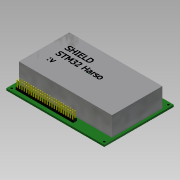
# Autodesk Inventor part: shieldstm
Saved by Autodesk Inventor 2015 SP1 (Build 190203100, 203)
## iProperties
Created: 2015-02-03
Part Number: shieldstm
Material: Generic
Document SubType Name: Modeling
Designer: Rafi Kurnia Putra
Density: 1 g/cm^3
Appearance: Smooth - Yellow
Mass: 140.996 g
Surface Area: 307.054 cm^2
Volume: 140.996 cm^3
Author: Rafi Kurnia Putra
Autodesk Inventor part; units mm, degrees
ref_plane "YZ Plane" through (0, 0, 0) normal (1, 0, 0) x (0, 1, 0)
ref_plane "XZ Plane" through (0, 0, 0) normal (0, 1, 0) x (-1, 0, 0)
ref_plane "XY Plane" through (0, 0, 0) normal (0, 0, 1) x (1, 0, 0)
sketch "Sketch1" plane through (0, 0, 0) normal (0, 1, 0) x (-1, 0, 0)
  line L0 (53.5965, 37.9955) -> (-53.5965, 37.9955)
  line L1 (-53.5965, 37.9955) -> (-53.5965, -37.9955)
  line L2 (-53.5965, -37.9955) -> (53.5965, -37.9955)
  line L3 (53.5965, -37.9955) -> (53.5965, 37.9955)
  line L4 (53.5965, 37.9955) -> (-53.5965, -37.9955) construction
  line L5 (-53.5965, 37.9955) -> (53.5965, -37.9955) construction
  circle A0 centre (50.5965, 34.9955) radius 1
  circle A1 centre (50.5965, -34.9955) radius 1
  circle A2 centre (-50.5965, 34.9955) radius 1
  circle A3 centre (-50.5965, -34.9955) radius 1
  line L6 (46.185, 33.9325) -> (45.392, 33.9325)
  line L7 (45.392, 33.9325) -> (45.392, 33.1485)
  line L8 (45.392, 33.1485) -> (46.185, 33.1485)
  line L9 (46.185, 33.1485) -> (46.185, 33.9325)
  line L10 (46.185, 33.9325) -> (45.392, 33.1485) construction
  line L11 (45.392, 33.9325) -> (46.185, 33.1485) construction
  line L12 (43.665, 33.9325) -> (42.872, 33.9325)
  line L13 (42.872, 33.9325) -> (42.872, 33.1485)
  line L14 (42.872, 33.1485) -> (43.665, 33.1485)
  line L15 (43.665, 33.1485) -> (43.665, 33.9325)
  line L16 (41.145, 33.9325) -> (40.352, 33.9325)
  line L17 (40.352, 33.9325) -> (40.352, 33.1485)
  line L18 (40.352, 33.1485) -> (41.145, 33.1485)
  line L19 (41.145, 33.1485) -> (41.145, 33.9325)
  line L20 (38.625, 33.9325) -> (37.832, 33.9325)
  line L21 (37.832, 33.9325) -> (37.832, 33.1485)
  line L22 (37.832, 33.1485) -> (38.625, 33.1485)
  line L23 (38.625, 33.1485) -> (38.625, 33.9325)
  line L24 (36.105, 33.9325) -> (35.312, 33.9325)
  line L25 (35.312, 33.9325) -> (35.312, 33.1485)
  line L26 (35.312, 33.1485) -> (36.105, 33.1485)
  line L27 (36.105, 33.1485) -> (36.105, 33.9325)
  line L28 (33.585, 33.9325) -> (32.792, 33.9325)
  line L29 (32.792, 33.9325) -> (32.792, 33.1485)
  line L30 (32.792, 33.1485) -> (33.585, 33.1485)
  line L31 (33.585, 33.1485) -> (33.585, 33.9325)
  line L32 (31.065, 33.9325) -> (30.272, 33.9325)
  line L33 (30.272, 33.9325) -> (30.272, 33.1485)
  line L34 (30.272, 33.1485) -> (31.065, 33.1485)
  line L35 (31.065, 33.1485) -> (31.065, 33.9325)
  line L36 (28.545, 33.9325) -> (27.752, 33.9325)
  line L37 (27.752, 33.9325) -> (27.752, 33.1485)
  line L38 (27.752, 33.1485) -> (28.545, 33.1485)
  line L39 (28.545, 33.1485) -> (28.545, 33.9325)
  line L40 (26.025, 33.9325) -> (25.232, 33.9325)
  line L41 (25.232, 33.9325) -> (25.232, 33.1485)
  line L42 (25.232, 33.1485) -> (26.025, 33.1485)
  line L43 (26.025, 33.1485) -> (26.025, 33.9325)
  line L44 (23.505, 33.9325) -> (22.712, 33.9325)
  line L45 (22.712, 33.9325) -> (22.712, 33.1485)
  line L46 (22.712, 33.1485) -> (23.505, 33.1485)
  line L47 (23.505, 33.1485) -> (23.505, 33.9325)
  line L48 (20.985, 33.9325) -> (20.192, 33.9325)
  line L49 (20.192, 33.9325) -> (20.192, 33.1485)
  line L50 (20.192, 33.1485) -> (20.985, 33.1485)
  line L51 (20.985, 33.1485) -> (20.985, 33.9325)
  line L52 (18.465, 33.9325) -> (17.672, 33.9325)
  line L53 (17.672, 33.9325) -> (17.672, 33.1485)
  line L54 (17.672, 33.1485) -> (18.465, 33.1485)
  line L55 (18.465, 33.1485) -> (18.465, 33.9325)
  line L56 (15.945, 33.9325) -> (15.152, 33.9325)
  line L57 (15.152, 33.9325) -> (15.152, 33.1485)
  line L58 (15.152, 33.1485) -> (15.945, 33.1485)
  line L59 (15.945, 33.1485) -> (15.945, 33.9325)
  line L60 (13.425, 33.9325) -> (12.632, 33.9325)
  line L61 (12.632, 33.9325) -> (12.632, 33.1485)
  line L62 (12.632, 33.1485) -> (13.425, 33.1485)
  line L63 (13.425, 33.1485) -> (13.425, 33.9325)
  line L64 (10.905, 33.9325) -> (10.112, 33.9325)
  line L65 (10.112, 33.9325) -> (10.112, 33.1485)
  line L66 (10.112, 33.1485) -> (10.905, 33.1485)
  line L67 (10.905, 33.1485) -> (10.905, 33.9325)
  line L68 (8.385, 33.9325) -> (7.592, 33.9325)
  line L69 (7.592, 33.9325) -> (7.592, 33.1485)
  line L70 (7.592, 33.1485) -> (8.385, 33.1485)
  line L71 (8.385, 33.1485) -> (8.385, 33.9325)
  line L72 (5.865, 33.9325) -> (5.072, 33.9325)
  line L73 (5.072, 33.9325) -> (5.072, 33.1485)
  line L74 (5.072, 33.1485) -> (5.865, 33.1485)
  line L75 (5.865, 33.1485) -> (5.865, 33.9325)
  line L76 (3.345, 33.9325) -> (2.552, 33.9325)
  line L77 (2.552, 33.9325) -> (2.552, 33.1485)
  line L78 (2.552, 33.1485) -> (3.345, 33.1485)
  line L79 (3.345, 33.1485) -> (3.345, 33.9325)
  line L80 (0.825, 33.9325) -> (0.032, 33.9325)
  line L81 (0.032, 33.9325) -> (0.032, 33.1485)
  line L82 (0.032, 33.1485) -> (0.825, 33.1485)
  line L83 (0.825, 33.1485) -> (0.825, 33.9325)
  line L84 (-1.695, 33.9325) -> (-2.488, 33.9325)
  line L85 (-2.488, 33.9325) -> (-2.488, 33.1485)
  line L86 (-2.488, 33.1485) -> (-1.695, 33.1485)
  line L87 (-1.695, 33.1485) -> (-1.695, 33.9325)
  line L88 (-4.215, 33.9325) -> (-5.008, 33.9325)
  line L89 (-5.008, 33.9325) -> (-5.008, 33.1485)
  line L90 (-5.008, 33.1485) -> (-4.215, 33.1485)
  line L91 (-4.215, 33.1485) -> (-4.215, 33.9325)
  line L92 (-6.735, 33.9325) -> (-7.528, 33.9325)
  line L93 (-7.528, 33.9325) -> (-7.528, 33.1485)
  line L94 (-7.528, 33.1485) -> (-6.735, 33.1485)
  line L95 (-6.735, 33.1485) -> (-6.735, 33.9325)
  line L96 (-9.255, 33.9325) -> (-10.048, 33.9325)
  line L97 (-10.048, 33.9325) -> (-10.048, 33.1485)
  line L98 (-10.048, 33.1485) -> (-9.255, 33.1485)
  line L99 (-9.255, 33.1485) -> (-9.255, 33.9325)
  line L100 (-11.775, 33.9325) -> (-12.568, 33.9325)
  line L101 (-12.568, 33.9325) -> (-12.568, 33.1485)
  line L102 (-12.568, 33.1485) -> (-11.775, 33.1485)
  line L103 (-11.775, 33.1485) -> (-11.775, 33.9325)
  line L104 (-14.295, 33.9325) -> (-15.088, 33.9325)
  line L105 (-15.088, 33.9325) -> (-15.088, 33.1485)
  line L106 (-15.088, 33.1485) -> (-14.295, 33.1485)
  line L107 (-14.295, 33.1485) -> (-14.295, 33.9325)
  line L108 (46.185, 31.4325) -> (45.392, 31.4325)
  line L109 (45.392, 31.4325) -> (45.392, 30.6485)
  line L110 (45.392, 30.6485) -> (46.185, 30.6485)
  line L111 (46.185, 30.6485) -> (46.185, 31.4325)
  line L112 (43.665, 31.4325) -> (42.872, 31.4325)
  line L113 (42.872, 31.4325) -> (42.872, 30.6485)
  line L114 (42.872, 30.6485) -> (43.665, 30.6485)
  line L115 (43.665, 30.6485) -> (43.665, 31.4325)
  line L116 (41.145, 31.4325) -> (40.352, 31.4325)
  line L117 (40.352, 31.4325) -> (40.352, 30.6485)
  line L118 (40.352, 30.6485) -> (41.145, 30.6485)
  line L119 (41.145, 30.6485) -> (41.145, 31.4325)
  line L120 (38.625, 31.4325) -> (37.832, 31.4325)
  line L121 (37.832, 31.4325) -> (37.832, 30.6485)
  line L122 (37.832, 30.6485) -> (38.625, 30.6485)
  line L123 (38.625, 30.6485) -> (38.625, 31.4325)
  line L124 (36.105, 31.4325) -> (35.312, 31.4325)
  line L125 (35.312, 31.4325) -> (35.312, 30.6485)
  line L126 (35.312, 30.6485) -> (36.105, 30.6485)
  line L127 (36.105, 30.6485) -> (36.105, 31.4325)
  line L128 (33.585, 31.4325) -> (32.792, 31.4325)
  line L129 (32.792, 31.4325) -> (32.792, 30.6485)
  line L130 (32.792, 30.6485) -> (33.585, 30.6485)
  line L131 (33.585, 30.6485) -> (33.585, 31.4325)
  line L132 (31.065, 31.4325) -> (30.272, 31.4325)
  line L133 (30.272, 31.4325) -> (30.272, 30.6485)
  line L134 (30.272, 30.6485) -> (31.065, 30.6485)
  line L135 (31.065, 30.6485) -> (31.065, 31.4325)
  line L136 (28.545, 31.4325) -> (27.752, 31.4325)
  line L137 (27.752, 31.4325) -> (27.752, 30.6485)
  line L138 (27.752, 30.6485) -> (28.545, 30.6485)
  line L139 (28.545, 30.6485) -> (28.545, 31.4325)
  line L140 (26.025, 31.4325) -> (25.232, 31.4325)
  line L141 (25.232, 31.4325) -> (25.232, 30.6485)
  line L142 (25.232, 30.6485) -> (26.025, 30.6485)
  line L143 (26.025, 30.6485) -> (26.025, 31.4325)
  line L144 (23.505, 31.4325) -> (22.712, 31.4325)
  line L145 (22.712, 31.4325) -> (22.712, 30.6485)
  line L146 (22.712, 30.6485) -> (23.505, 30.6485)
  line L147 (23.505, 30.6485) -> (23.505, 31.4325)
  line L148 (20.985, 31.4325) -> (20.192, 31.4325)
  line L149 (20.192, 31.4325) -> (20.192, 30.6485)
  line L150 (20.192, 30.6485) -> (20.985, 30.6485)
  line L151 (20.985, 30.6485) -> (20.985, 31.4325)
  line L152 (18.465, 31.4325) -> (17.672, 31.4325)
  line L153 (17.672, 31.4325) -> (17.672, 30.6485)
  line L154 (17.672, 30.6485) -> (18.465, 30.6485)
  line L155 (18.465, 30.6485) -> (18.465, 31.4325)
  line L156 (15.945, 31.4325) -> (15.152, 31.4325)
  line L157 (15.152, 31.4325) -> (15.152, 30.6485)
  line L158 (15.152, 30.6485) -> (15.945, 30.6485)
  line L159 (15.945, 30.6485) -> (15.945, 31.4325)
  line L160 (13.425, 31.4325) -> (12.632, 31.4325)
  line L161 (12.632, 31.4325) -> (12.632, 30.6485)
  line L162 (12.632, 30.6485) -> (13.425, 30.6485)
  line L163 (13.425, 30.6485) -> (13.425, 31.4325)
  line L164 (10.905, 31.4325) -> (10.112, 31.4325)
  line L165 (10.112, 31.4325) -> (10.112, 30.6485)
  line L166 (10.112, 30.6485) -> (10.905, 30.6485)
  line L167 (10.905, 30.6485) -> (10.905, 31.4325)
  line L168 (8.385, 31.4325) -> (7.592, 31.4325)
  line L169 (7.592, 31.4325) -> (7.592, 30.6485)
  line L170 (7.592, 30.6485) -> (8.385, 30.6485)
  line L171 (8.385, 30.6485) -> (8.385, 31.4325)
  line L172 (5.865, 31.4325) -> (5.072, 31.4325)
  line L173 (5.072, 31.4325) -> (5.072, 30.6485)
  line L174 (5.072, 30.6485) -> (5.865, 30.6485)
  line L175 (5.865, 30.6485) -> (5.865, 31.4325)
  line L176 (3.345, 31.4325) -> (2.552, 31.4325)
  line L177 (2.552, 31.4325) -> (2.552, 30.6485)
  line L178 (2.552, 30.6485) -> (3.345, 30.6485)
  line L179 (3.345, 30.6485) -> (3.345, 31.4325)
  line L180 (0.825, 31.4325) -> (0.032, 31.4325)
  line L181 (0.032, 31.4325) -> (0.032, 30.6485)
  line L182 (0.032, 30.6485) -> (0.825, 30.6485)
  line L183 (0.825, 30.6485) -> (0.825, 31.4325)
  line L184 (-1.695, 31.4325) -> (-2.488, 31.4325)
  line L185 (-2.488, 31.4325) -> (-2.488, 30.6485)
  line L186 (-2.488, 30.6485) -> (-1.695, 30.6485)
  line L187 (-1.695, 30.6485) -> (-1.695, 31.4325)
  line L188 (-4.215, 31.4325) -> (-5.008, 31.4325)
  line L189 (-5.008, 31.4325) -> (-5.008, 30.6485)
  line L190 (-5.008, 30.6485) -> (-4.215, 30.6485)
  line L191 (-4.215, 30.6485) -> (-4.215, 31.4325)
  line L192 (-6.735, 31.4325) -> (-7.528, 31.4325)
  line L193 (-7.528, 31.4325) -> (-7.528, 30.6485)
  line L194 (-7.528, 30.6485) -> (-6.735, 30.6485)
  line L195 (-6.735, 30.6485) -> (-6.735, 31.4325)
  line L196 (-9.255, 31.4325) -> (-10.048, 31.4325)
  line L197 (-10.048, 31.4325) -> (-10.048, 30.6485)
  line L198 (-10.048, 30.6485) -> (-9.255, 30.6485)
  line L199 (-9.255, 30.6485) -> (-9.255, 31.4325)
  line L200 (-11.775, 31.4325) -> (-12.568, 31.4325)
  line L201 (-12.568, 31.4325) -> (-12.568, 30.6485)
  line L202 (-12.568, 30.6485) -> (-11.775, 30.6485)
  line L203 (-11.775, 30.6485) -> (-11.775, 31.4325)
  line L204 (-14.295, 31.4325) -> (-15.088, 31.4325)
  line L205 (-15.088, 31.4325) -> (-15.088, 30.6485)
  line L206 (-15.088, 30.6485) -> (-14.295, 30.6485)
  line L207 (-14.295, 30.6485) -> (-14.295, 31.4325)
  line L208 (45.392, 27.0175) -> (46.185, 27.0175)
  line L209 (46.185, 27.0175) -> (46.185, 26.2335)
  line L210 (46.185, 26.2335) -> (45.392, 26.2335)
  line L211 (45.392, 26.2335) -> (45.392, 27.0175)
  line L212 (45.392, 27.0175) -> (46.185, 26.2335) construction
  line L213 (46.185, 27.0175) -> (45.392, 26.2335) construction
  line L214 (42.872, 27.0175) -> (43.665, 27.0175)
  line L215 (43.665, 27.0175) -> (43.665, 26.2335)
  line L216 (43.665, 26.2335) -> (42.872, 26.2335)
  line L217 (42.872, 26.2335) -> (42.872, 27.0175)
  line L218 (40.352, 27.0175) -> (41.145, 27.0175)
  line L219 (41.145, 27.0175) -> (41.145, 26.2335)
  line L220 (41.145, 26.2335) -> (40.352, 26.2335)
  line L221 (40.352, 26.2335) -> (40.352, 27.0175)
  line L222 (37.832, 27.0175) -> (38.625, 27.0175)
  line L223 (38.625, 27.0175) -> (38.625, 26.2335)
  line L224 (38.625, 26.2335) -> (37.832, 26.2335)
  line L225 (37.832, 26.2335) -> (37.832, 27.0175)
  line L226 (35.312, 27.0175) -> (36.105, 27.0175)
  line L227 (36.105, 27.0175) -> (36.105, 26.2335)
  line L228 (36.105, 26.2335) -> (35.312, 26.2335)
  line L229 (35.312, 26.2335) -> (35.312, 27.0175)
  line L230 (32.792, 27.0175) -> (33.585, 27.0175)
  line L231 (33.585, 27.0175) -> (33.585, 26.2335)
  line L232 (33.585, 26.2335) -> (32.792, 26.2335)
  line L233 (32.792, 26.2335) -> (32.792, 27.0175)
  line L234 (30.272, 27.0175) -> (31.065, 27.0175)
  line L235 (31.065, 27.0175) -> (31.065, 26.2335)
  line L236 (31.065, 26.2335) -> (30.272, 26.2335)
  line L237 (30.272, 26.2335) -> (30.272, 27.0175)
  line L238 (27.752, 27.0175) -> (28.545, 27.0175)
  line L239 (28.545, 27.0175) -> (28.545, 26.2335)
  line L240 (28.545, 26.2335) -> (27.752, 26.2335)
  line L241 (27.752, 26.2335) -> (27.752, 27.0175)
  line L242 (25.232, 27.0175) -> (26.025, 27.0175)
  line L243 (26.025, 27.0175) -> (26.025, 26.2335)
  line L244 (26.025, 26.2335) -> (25.232, 26.2335)
  line L245 (25.232, 26.2335) -> (25.232, 27.0175)
  line L246 (22.712, 27.0175) -> (23.505, 27.0175)
  line L247 (23.505, 27.0175) -> (23.505, 26.2335)
  line L248 (23.505, 26.2335) -> (22.712, 26.2335)
  line L249 (22.712, 26.2335) -> (22.712, 27.0175)
  line L250 (20.192, 27.0175) -> (20.985, 27.0175)
  line L251 (20.985, 27.0175) -> (20.985, 26.2335)
  line L252 (20.985, 26.2335) -> (20.192, 26.2335)
  line L253 (20.192, 26.2335) -> (20.192, 27.0175)
  line L254 (17.672, 27.0175) -> (18.465, 27.0175)
  line L255 (18.465, 27.0175) -> (18.465, 26.2335)
  line L256 (18.465, 26.2335) -> (17.672, 26.2335)
  line L257 (17.672, 26.2335) -> (17.672, 27.0175)
  line L258 (15.152, 27.0175) -> (15.945, 27.0175)
  line L259 (15.945, 27.0175) -> (15.945, 26.2335)
  line L260 (15.945, 26.2335) -> (15.152, 26.2335)
  line L261 (15.152, 26.2335) -> (15.152, 27.0175)
  line L262 (12.632, 27.0175) -> (13.425, 27.0175)
  line L263 (13.425, 27.0175) -> (13.425, 26.2335)
  line L264 (13.425, 26.2335) -> (12.632, 26.2335)
  line L265 (12.632, 26.2335) -> (12.632, 27.0175)
  line L266 (10.112, 27.0175) -> (10.905, 27.0175)
  line L267 (10.905, 27.0175) -> (10.905, 26.2335)
  line L268 (10.905, 26.2335) -> (10.112, 26.2335)
  line L269 (10.112, 26.2335) -> (10.112, 27.0175)
  line L270 (7.592, 27.0175) -> (8.385, 27.0175)
  line L271 (8.385, 27.0175) -> (8.385, 26.2335)
  line L272 (8.385, 26.2335) -> (7.592, 26.2335)
  line L273 (7.592, 26.2335) -> (7.592, 27.0175)
  line L274 (5.072, 27.0175) -> (5.865, 27.0175)
  line L275 (5.865, 27.0175) -> (5.865, 26.2335)
  line L276 (5.865, 26.2335) -> (5.072, 26.2335)
  line L277 (5.072, 26.2335) -> (5.072, 27.0175)
  line L278 (2.552, 27.0175) -> (3.345, 27.0175)
  line L279 (3.345, 27.0175) -> (3.345, 26.2335)
  line L280 (3.345, 26.2335) -> (2.552, 26.2335)
  line L281 (2.552, 26.2335) -> (2.552, 27.0175)
  line L282 (0.032, 27.0175) -> (0.825, 27.0175)
  line L283 (0.825, 27.0175) -> (0.825, 26.2335)
  line L284 (0.825, 26.2335) -> (0.032, 26.2335)
  line L285 (0.032, 26.2335) -> (0.032, 27.0175)
  line L286 (-2.488, 27.0175) -> (-1.695, 27.0175)
  line L287 (-1.695, 27.0175) -> (-1.695, 26.2335)
  line L288 (-1.695, 26.2335) -> (-2.488, 26.2335)
  line L289 (-2.488, 26.2335) -> (-2.488, 27.0175)
  line L290 (-5.008, 27.0175) -> (-4.215, 27.0175)
  line L291 (-4.215, 27.0175) -> (-4.215, 26.2335)
  line L292 (-4.215, 26.2335) -> (-5.008, 26.2335)
  line L293 (-5.008, 26.2335) -> (-5.008, 27.0175)
  line L294 (-7.528, 27.0175) -> (-6.735, 27.0175)
  line L295 (-6.735, 27.0175) -> (-6.735, 26.2335)
  line L296 (-6.735, 26.2335) -> (-7.528, 26.2335)
  line L297 (-7.528, 26.2335) -> (-7.528, 27.0175)
  line L298 (-10.048, 27.0175) -> (-9.255, 27.0175)
  line L299 (-9.255, 27.0175) -> (-9.255, 26.2335)
  line L300 (-9.255, 26.2335) -> (-10.048, 26.2335)
  line L301 (-10.048, 26.2335) -> (-10.048, 27.0175)
  line L302 (-12.568, 27.0175) -> (-11.775, 27.0175)
  line L303 (-11.775, 27.0175) -> (-11.775, 26.2335)
  line L304 (-11.775, 26.2335) -> (-12.568, 26.2335)
  line L305 (-12.568, 26.2335) -> (-12.568, 27.0175)
  line L306 (-15.088, 27.0175) -> (-14.295, 27.0175)
  line L307 (-14.295, 27.0175) -> (-14.295, 26.2335)
  line L308 (-14.295, 26.2335) -> (-15.088, 26.2335)
  line L309 (-15.088, 26.2335) -> (-15.088, 27.0175)
  line L310 (45.392, 24.5175) -> (46.185, 24.5175)
  line L311 (46.185, 24.5175) -> (46.185, 23.7335)
  line L312 (46.185, 23.7335) -> (45.392, 23.7335)
  line L313 (45.392, 23.7335) -> (45.392, 24.5175)
  line L314 (42.872, 24.5175) -> (43.665, 24.5175)
  line L315 (43.665, 24.5175) -> (43.665, 23.7335)
  line L316 (43.665, 23.7335) -> (42.872, 23.7335)
  line L317 (42.872, 23.7335) -> (42.872, 24.5175)
  line L318 (40.352, 24.5175) -> (41.145, 24.5175)
  line L319 (41.145, 24.5175) -> (41.145, 23.7335)
  line L320 (41.145, 23.7335) -> (40.352, 23.7335)
  line L321 (40.352, 23.7335) -> (40.352, 24.5175)
  line L322 (37.832, 24.5175) -> (38.625, 24.5175)
  line L323 (38.625, 24.5175) -> (38.625, 23.7335)
  line L324 (38.625, 23.7335) -> (37.832, 23.7335)
  line L325 (37.832, 23.7335) -> (37.832, 24.5175)
  line L326 (35.312, 24.5175) -> (36.105, 24.5175)
  line L327 (36.105, 24.5175) -> (36.105, 23.7335)
  line L328 (36.105, 23.7335) -> (35.312, 23.7335)
  line L329 (35.312, 23.7335) -> (35.312, 24.5175)
  line L330 (32.792, 24.5175) -> (33.585, 24.5175)
  line L331 (33.585, 24.5175) -> (33.585, 23.7335)
  line L332 (33.585, 23.7335) -> (32.792, 23.7335)
  line L333 (32.792, 23.7335) -> (32.792, 24.5175)
  line L334 (30.272, 24.5175) -> (31.065, 24.5175)
  line L335 (31.065, 24.5175) -> (31.065, 23.7335)
  line L336 (31.065, 23.7335) -> (30.272, 23.7335)
  line L337 (30.272, 23.7335) -> (30.272, 24.5175)
  line L338 (27.752, 24.5175) -> (28.545, 24.5175)
  line L339 (28.545, 24.5175) -> (28.545, 23.7335)
  line L340 (28.545, 23.7335) -> (27.752, 23.7335)
  line L341 (27.752, 23.7335) -> (27.752, 24.5175)
  line L342 (25.232, 24.5175) -> (26.025, 24.5175)
  line L343 (26.025, 24.5175) -> (26.025, 23.7335)
  line L344 (26.025, 23.7335) -> (25.232, 23.7335)
  line L345 (25.232, 23.7335) -> (25.232, 24.5175)
  line L346 (22.712, 24.5175) -> (23.505, 24.5175)
  line L347 (23.505, 24.5175) -> (23.505, 23.7335)
  line L348 (23.505, 23.7335) -> (22.712, 23.7335)
  line L349 (22.712, 23.7335) -> (22.712, 24.5175)
  line L350 (20.192, 24.5175) -> (20.985, 24.5175)
  line L351 (20.985, 24.5175) -> (20.985, 23.7335)
  line L352 (20.985, 23.7335) -> (20.192, 23.7335)
  line L353 (20.192, 23.7335) -> (20.192, 24.5175)
  line L354 (17.672, 24.5175) -> (18.465, 24.5175)
  line L355 (18.465, 24.5175) -> (18.465, 23.7335)
  line L356 (18.465, 23.7335) -> (17.672, 23.7335)
  line L357 (17.672, 23.7335) -> (17.672, 24.5175)
  line L358 (15.152, 24.5175) -> (15.945, 24.5175)
  line L359 (15.945, 24.5175) -> (15.945, 23.7335)
  line L360 (15.945, 23.7335) -> (15.152, 23.7335)
  line L361 (15.152, 23.7335) -> (15.152, 24.5175)
  line L362 (12.632, 24.5175) -> (13.425, 24.5175)
  line L363 (13.425, 24.5175) -> (13.425, 23.7335)
  line L364 (13.425, 23.7335) -> (12.632, 23.7335)
  line L365 (12.632, 23.7335) -> (12.632, 24.5175)
  line L366 (10.112, 24.5175) -> (10.905, 24.5175)
  line L367 (10.905, 24.5175) -> (10.905, 23.7335)
  line L368 (10.905, 23.7335) -> (10.112, 23.7335)
  line L369 (10.112, 23.7335) -> (10.112, 24.5175)
  line L370 (7.592, 24.5175) -> (8.385, 24.5175)
  line L371 (8.385, 24.5175) -> (8.385, 23.7335)
  line L372 (8.385, 23.7335) -> (7.592, 23.7335)
  line L373 (7.592, 23.7335) -> (7.592, 24.5175)
  line L374 (5.072, 24.5175) -> (5.865, 24.5175)
  line L375 (5.865, 24.5175) -> (5.865, 23.7335)
  line L376 (5.865, 23.7335) -> (5.072, 23.7335)
  line L377 (5.072, 23.7335) -> (5.072, 24.5175)
  line L378 (2.552, 24.5175) -> (3.345, 24.5175)
  line L379 (3.345, 24.5175) -> (3.345, 23.7335)
  line L380 (3.345, 23.7335) -> (2.552, 23.7335)
  line L381 (2.552, 23.7335) -> (2.552, 24.5175)
  line L382 (0.032, 24.5175) -> (0.825, 24.5175)
  line L383 (0.825, 24.5175) -> (0.825, 23.7335)
  line L384 (0.825, 23.7335) -> (0.032, 23.7335)
  line L385 (0.032, 23.7335) -> (0.032, 24.5175)
  line L386 (-2.488, 24.5175) -> (-1.695, 24.5175)
  line L387 (-1.695, 24.5175) -> (-1.695, 23.7335)
  line L388 (-1.695, 23.7335) -> (-2.488, 23.7335)
  line L389 (-2.488, 23.7335) -> (-2.488, 24.5175)
  line L390 (-5.008, 24.5175) -> (-4.215, 24.5175)
  line L391 (-4.215, 24.5175) -> (-4.215, 23.7335)
  line L392 (-4.215, 23.7335) -> (-5.008, 23.7335)
  line L393 (-5.008, 23.7335) -> (-5.008, 24.5175)
  line L394 (-7.528, 24.5175) -> (-6.735, 24.5175)
  line L395 (-6.735, 24.5175) -> (-6.735, 23.7335)
  line L396 (-6.735, 23.7335) -> (-7.528, 23.7335)
  line L397 (-7.528, 23.7335) -> (-7.528, 24.5175)
  line L398 (-10.048, 24.5175) -> (-9.255, 24.5175)
  line L399 (-9.255, 24.5175) -> (-9.255, 23.7335)
  line L400 (-9.255, 23.7335) -> (-10.048, 23.7335)
  line L401 (-10.048, 23.7335) -> (-10.048, 24.5175)
  line L402 (-12.568, 24.5175) -> (-11.775, 24.5175)
  line L403 (-11.775, 24.5175) -> (-11.775, 23.7335)
  line L404 (-11.775, 23.7335) -> (-12.568, 23.7335)
  line L405 (-12.568, 23.7335) -> (-12.568, 24.5175)
  line L406 (-15.088, 24.5175) -> (-14.295, 24.5175)
  line L407 (-14.295, 24.5175) -> (-14.295, 23.7335)
  line L408 (-14.295, 23.7335) -> (-15.088, 23.7335)
  line L409 (-15.088, 23.7335) -> (-15.088, 24.5175)
  line L410 (47.0585, 27.8955) -> (-15.9615, 27.8955)
  line L411 (-15.9615, 27.8955) -> (-15.9615, 22.8555)
  line L412 (-15.9615, 22.8555) -> (47.0585, 22.8555)
  line L413 (47.0585, 22.8555) -> (47.0585, 27.8955)
  line L414 (53.5965, -37.9955) -> (-53.5965, 37.9955) construction
  line L415 (-53.5965, -37.9955) -> (53.5965, 37.9955) construction
  line L416 (46.185, -33.9325) -> (45.392, -33.9325)
  line L417 (45.392, -33.9325) -> (45.392, -33.1485)
  line L418 (45.392, -33.1485) -> (46.185, -33.1485)
  line L419 (46.185, -33.1485) -> (46.185, -33.9325)
  line L420 (46.185, -33.9325) -> (45.392, -33.1485) construction
  line L421 (45.392, -33.9325) -> (46.185, -33.1485) construction
  line L422 (42.872, -33.9325) -> (42.872, -33.1485)
  line L423 (43.665, -33.9325) -> (42.872, -33.9325)
  line L424 (43.665, -33.1485) -> (43.665, -33.9325)
  line L425 (42.872, -33.1485) -> (43.665, -33.1485)
  line L426 (40.352, -33.9325) -> (40.352, -33.1485)
  line L427 (41.145, -33.9325) -> (40.352, -33.9325)
  line L428 (41.145, -33.1485) -> (41.145, -33.9325)
  line L429 (40.352, -33.1485) -> (41.145, -33.1485)
  line L430 (37.832, -33.9325) -> (37.832, -33.1485)
  line L431 (38.625, -33.9325) -> (37.832, -33.9325)
  line L432 (38.625, -33.1485) -> (38.625, -33.9325)
  line L433 (37.832, -33.1485) -> (38.625, -33.1485)
  line L434 (35.312, -33.9325) -> (35.312, -33.1485)
  line L435 (36.105, -33.9325) -> (35.312, -33.9325)
  line L436 (36.105, -33.1485) -> (36.105, -33.9325)
  line L437 (35.312, -33.1485) -> (36.105, -33.1485)
  line L438 (32.792, -33.9325) -> (32.792, -33.1485)
  line L439 (33.585, -33.9325) -> (32.792, -33.9325)
  line L440 (33.585, -33.1485) -> (33.585, -33.9325)
  line L441 (32.792, -33.1485) -> (33.585, -33.1485)
  line L442 (30.272, -33.9325) -> (30.272, -33.1485)
  line L443 (31.065, -33.9325) -> (30.272, -33.9325)
  line L444 (31.065, -33.1485) -> (31.065, -33.9325)
  line L445 (30.272, -33.1485) -> (31.065, -33.1485)
  line L446 (27.752, -33.9325) -> (27.752, -33.1485)
  line L447 (28.545, -33.9325) -> (27.752, -33.9325)
  line L448 (28.545, -33.1485) -> (28.545, -33.9325)
  line L449 (27.752, -33.1485) -> (28.545, -33.1485)
  line L450 (25.232, -33.9325) -> (25.232, -33.1485)
  line L451 (26.025, -33.9325) -> (25.232, -33.9325)
  line L452 (26.025, -33.1485) -> (26.025, -33.9325)
  line L453 (25.232, -33.1485) -> (26.025, -33.1485)
  line L454 (22.712, -33.9325) -> (22.712, -33.1485)
  line L455 (23.505, -33.9325) -> (22.712, -33.9325)
  line L456 (23.505, -33.1485) -> (23.505, -33.9325)
  line L457 (22.712, -33.1485) -> (23.505, -33.1485)
  line L458 (20.192, -33.9325) -> (20.192, -33.1485)
  line L459 (20.985, -33.9325) -> (20.192, -33.9325)
  line L460 (20.985, -33.1485) -> (20.985, -33.9325)
  line L461 (20.192, -33.1485) -> (20.985, -33.1485)
  line L462 (17.672, -33.9325) -> (17.672, -33.1485)
  line L463 (18.465, -33.9325) -> (17.672, -33.9325)
  line L464 (18.465, -33.1485) -> (18.465, -33.9325)
  line L465 (17.672, -33.1485) -> (18.465, -33.1485)
  line L466 (15.152, -33.9325) -> (15.152, -33.1485)
  line L467 (15.945, -33.9325) -> (15.152, -33.9325)
  line L468 (15.945, -33.1485) -> (15.945, -33.9325)
  line L469 (15.152, -33.1485) -> (15.945, -33.1485)
  line L470 (12.632, -33.9325) -> (12.632, -33.1485)
  line L471 (13.425, -33.9325) -> (12.632, -33.9325)
  line L472 (13.425, -33.1485) -> (13.425, -33.9325)
  line L473 (12.632, -33.1485) -> (13.425, -33.1485)
  line L474 (10.112, -33.9325) -> (10.112, -33.1485)
  line L475 (10.905, -33.9325) -> (10.112, -33.9325)
  line L476 (10.905, -33.1485) -> (10.905, -33.9325)
  line L477 (10.112, -33.1485) -> (10.905, -33.1485)
  line L478 (7.592, -33.9325) -> (7.592, -33.1485)
  line L479 (8.385, -33.9325) -> (7.592, -33.9325)
  line L480 (8.385, -33.1485) -> (8.385, -33.9325)
  line L481 (7.592, -33.1485) -> (8.385, -33.1485)
  line L482 (5.072, -33.9325) -> (5.072, -33.1485)
  line L483 (5.865, -33.9325) -> (5.072, -33.9325)
  line L484 (5.865, -33.1485) -> (5.865, -33.9325)
  line L485 (5.072, -33.1485) -> (5.865, -33.1485)
  line L486 (2.552, -33.9325) -> (2.552, -33.1485)
  line L487 (3.345, -33.9325) -> (2.552, -33.9325)
  line L488 (3.345, -33.1485) -> (3.345, -33.9325)
  line L489 (2.552, -33.1485) -> (3.345, -33.1485)
  line L490 (0.032, -33.9325) -> (0.032, -33.1485)
  line L491 (0.825, -33.9325) -> (0.032, -33.9325)
  line L492 (0.825, -33.1485) -> (0.825, -33.9325)
  line L493 (0.032, -33.1485) -> (0.825, -33.1485)
  line L494 (-2.488, -33.9325) -> (-2.488, -33.1485)
  line L495 (-1.695, -33.9325) -> (-2.488, -33.9325)
  line L496 (-1.695, -33.1485) -> (-1.695, -33.9325)
  line L497 (-2.488, -33.1485) -> (-1.695, -33.1485)
  line L498 (-5.008, -33.9325) -> (-5.008, -33.1485)
  line L499 (-4.215, -33.9325) -> (-5.008, -33.9325)
  line L500 (-4.215, -33.1485) -> (-4.215, -33.9325)
  line L501 (-5.008, -33.1485) -> (-4.215, -33.1485)
  line L502 (-7.528, -33.9325) -> (-7.528, -33.1485)
  line L503 (-6.735, -33.9325) -> (-7.528, -33.9325)
  line L504 (-6.735, -33.1485) -> (-6.735, -33.9325)
  line L505 (-7.528, -33.1485) -> (-6.735, -33.1485)
  line L506 (-10.048, -33.9325) -> (-10.048, -33.1485)
  line L507 (-9.255, -33.9325) -> (-10.048, -33.9325)
  line L508 (-9.255, -33.1485) -> (-9.255, -33.9325)
  line L509 (-10.048, -33.1485) -> (-9.255, -33.1485)
  line L510 (-12.568, -33.9325) -> (-12.568, -33.1485)
  line L511 (-11.775, -33.9325) -> (-12.568, -33.9325)
  line L512 (-11.775, -33.1485) -> (-11.775, -33.9325)
  line L513 (-12.568, -33.1485) -> (-11.775, -33.1485)
  line L514 (-15.088, -33.9325) -> (-15.088, -33.1485)
  line L515 (-14.295, -33.9325) -> (-15.088, -33.9325)
  line L516 (-14.295, -33.1485) -> (-14.295, -33.9325)
  line L517 (-15.088, -33.1485) -> (-14.295, -33.1485)
  line L518 (45.392, -31.4325) -> (45.392, -30.6485)
  line L519 (46.185, -31.4325) -> (45.392, -31.4325)
  line L520 (46.185, -30.6485) -> (46.185, -31.4325)
  line L521 (45.392, -30.6485) -> (46.185, -30.6485)
  line L522 (42.872, -31.4325) -> (42.872, -30.6485)
  line L523 (43.665, -31.4325) -> (42.872, -31.4325)
  line L524 (43.665, -30.6485) -> (43.665, -31.4325)
  line L525 (42.872, -30.6485) -> (43.665, -30.6485)
  line L526 (40.352, -31.4325) -> (40.352, -30.6485)
  line L527 (41.145, -31.4325) -> (40.352, -31.4325)
  line L528 (41.145, -30.6485) -> (41.145, -31.4325)
  line L529 (40.352, -30.6485) -> (41.145, -30.6485)
  line L530 (37.832, -31.4325) -> (37.832, -30.6485)
  line L531 (38.625, -31.4325) -> (37.832, -31.4325)
  line L532 (38.625, -30.6485) -> (38.625, -31.4325)
  line L533 (37.832, -30.6485) -> (38.625, -30.6485)
  line L534 (35.312, -31.4325) -> (35.312, -30.6485)
  line L535 (36.105, -31.4325) -> (35.312, -31.4325)
  line L536 (36.105, -30.6485) -> (36.105, -31.4325)
  line L537 (35.312, -30.6485) -> (36.105, -30.6485)
  line L538 (32.792, -31.4325) -> (32.792, -30.6485)
  line L539 (33.585, -31.4325) -> (32.792, -31.4325)
  line L540 (33.585, -30.6485) -> (33.585, -31.4325)
  line L541 (32.792, -30.6485) -> (33.585, -30.6485)
  line L542 (30.272, -31.4325) -> (30.272, -30.6485)
  line L543 (31.065, -31.4325) -> (30.272, -31.4325)
  line L544 (31.065, -30.6485) -> (31.065, -31.4325)
  line L545 (30.272, -30.6485) -> (31.065, -30.6485)
  line L546 (27.752, -31.4325) -> (27.752, -30.6485)
  line L547 (28.545, -31.4325) -> (27.752, -31.4325)
  line L548 (28.545, -30.6485) -> (28.545, -31.4325)
  line L549 (27.752, -30.6485) -> (28.545, -30.6485)
  line L550 (25.232, -31.4325) -> (25.232, -30.6485)
  line L551 (26.025, -31.4325) -> (25.232, -31.4325)
  line L552 (26.025, -30.6485) -> (26.025, -31.4325)
  line L553 (25.232, -30.6485) -> (26.025, -30.6485)
  line L554 (22.712, -31.4325) -> (22.712, -30.6485)
  line L555 (23.505, -31.4325) -> (22.712, -31.4325)
  line L556 (23.505, -30.6485) -> (23.505, -31.4325)
  line L557 (22.712, -30.6485) -> (23.505, -30.6485)
  line L558 (20.192, -31.4325) -> (20.192, -30.6485)
  line L559 (20.985, -31.4325) -> (20.192, -31.4325)
  line L560 (20.985, -30.6485) -> (20.985, -31.4325)
  line L561 (20.192, -30.6485) -> (20.985, -30.6485)
  line L562 (17.672, -31.4325) -> (17.672, -30.6485)
  line L563 (18.465, -31.4325) -> (17.672, -31.4325)
  line L564 (18.465, -30.6485) -> (18.465, -31.4325)
  line L565 (17.672, -30.6485) -> (18.465, -30.6485)
  line L566 (15.152, -31.4325) -> (15.152, -30.6485)
  line L567 (15.945, -31.4325) -> (15.152, -31.4325)
  line L568 (15.945, -30.6485) -> (15.945, -31.4325)
  line L569 (15.152, -30.6485) -> (15.945, -30.6485)
  line L570 (12.632, -31.4325) -> (12.632, -30.6485)
  line L571 (13.425, -31.4325) -> (12.632, -31.4325)
  line L572 (13.425, -30.6485) -> (13.425, -31.4325)
  line L573 (12.632, -30.6485) -> (13.425, -30.6485)
  line L574 (10.112, -31.4325) -> (10.112, -30.6485)
  line L575 (10.905, -31.4325) -> (10.112, -31.4325)
  line L576 (10.905, -30.6485) -> (10.905, -31.4325)
  line L577 (10.112, -30.6485) -> (10.905, -30.6485)
  line L578 (7.592, -31.4325) -> (7.592, -30.6485)
  line L579 (8.385, -31.4325) -> (7.592, -31.4325)
  line L580 (8.385, -30.6485) -> (8.385, -31.4325)
  line L581 (7.592, -30.6485) -> (8.385, -30.6485)
  line L582 (5.072, -31.4325) -> (5.072, -30.6485)
  line L583 (5.865, -31.4325) -> (5.072, -31.4325)
  line L584 (5.865, -30.6485) -> (5.865, -31.4325)
  line L585 (5.072, -30.6485) -> (5.865, -30.6485)
  line L586 (2.552, -31.4325) -> (2.552, -30.6485)
  line L587 (3.345, -31.4325) -> (2.552, -31.4325)
  line L588 (3.345, -30.6485) -> (3.345, -31.4325)
  line L589 (2.552, -30.6485) -> (3.345, -30.6485)
  line L590 (0.032, -31.4325) -> (0.032, -30.6485)
  line L591 (0.825, -31.4325) -> (0.032, -31.4325)
  line L592 (0.825, -30.6485) -> (0.825, -31.4325)
  line L593 (0.032, -30.6485) -> (0.825, -30.6485)
  line L594 (-2.488, -31.4325) -> (-2.488, -30.6485)
  line L595 (-1.695, -31.4325) -> (-2.488, -31.4325)
  line L596 (-1.695, -30.6485) -> (-1.695, -31.4325)
  line L597 (-2.488, -30.6485) -> (-1.695, -30.6485)
  line L598 (-5.008, -31.4325) -> (-5.008, -30.6485)
  line L599 (-4.215, -31.4325) -> (-5.008, -31.4325)
  line L600 (-4.215, -30.6485) -> (-4.215, -31.4325)
  line L601 (-5.008, -30.6485) -> (-4.215, -30.6485)
  line L602 (-7.528, -31.4325) -> (-7.528, -30.6485)
  line L603 (-6.735, -31.4325) -> (-7.528, -31.4325)
  line L604 (-6.735, -30.6485) -> (-6.735, -31.4325)
  line L605 (-7.528, -30.6485) -> (-6.735, -30.6485)
  line L606 (-10.048, -31.4325) -> (-10.048, -30.6485)
  line L607 (-9.255, -31.4325) -> (-10.048, -31.4325)
  line L608 (-9.255, -30.6485) -> (-9.255, -31.4325)
  line L609 (-10.048, -30.6485) -> (-9.255, -30.6485)
  line L610 (-12.568, -31.4325) -> (-12.568, -30.6485)
  line L611 (-11.775, -31.4325) -> (-12.568, -31.4325)
  line L612 (-11.775, -30.6485) -> (-11.775, -31.4325)
  line L613 (-12.568, -30.6485) -> (-11.775, -30.6485)
  line L614 (-15.088, -31.4325) -> (-15.088, -30.6485)
  line L615 (-14.295, -31.4325) -> (-15.088, -31.4325)
  line L616 (-14.295, -30.6485) -> (-14.295, -31.4325)
  line L617 (-15.088, -30.6485) -> (-14.295, -30.6485)
  line L618 (45.392, -27.0175) -> (46.185, -27.0175)
  line L619 (46.185, -27.0175) -> (46.185, -26.2335)
  line L620 (46.185, -26.2335) -> (45.392, -26.2335)
  line L621 (45.392, -26.2335) -> (45.392, -27.0175)
  line L622 (45.392, -27.0175) -> (46.185, -26.2335) construction
  line L623 (46.185, -27.0175) -> (45.392, -26.2335) construction
  line L624 (42.872, -26.2335) -> (42.872, -27.0175)
  line L625 (43.665, -26.2335) -> (42.872, -26.2335)
  line L626 (43.665, -27.0175) -> (43.665, -26.2335)
  line L627 (42.872, -27.0175) -> (43.665, -27.0175)
  line L628 (40.352, -26.2335) -> (40.352, -27.0175)
  line L629 (41.145, -26.2335) -> (40.352, -26.2335)
  line L630 (41.145, -27.0175) -> (41.145, -26.2335)
  line L631 (40.352, -27.0175) -> (41.145, -27.0175)
  line L632 (37.832, -26.2335) -> (37.832, -27.0175)
  line L633 (38.625, -26.2335) -> (37.832, -26.2335)
  line L634 (38.625, -27.0175) -> (38.625, -26.2335)
  line L635 (37.832, -27.0175) -> (38.625, -27.0175)
  line L636 (35.312, -26.2335) -> (35.312, -27.0175)
  line L637 (36.105, -26.2335) -> (35.312, -26.2335)
  line L638 (36.105, -27.0175) -> (36.105, -26.2335)
  line L639 (35.312, -27.0175) -> (36.105, -27.0175)
  line L640 (32.792, -26.2335) -> (32.792, -27.0175)
  line L641 (33.585, -26.2335) -> (32.792, -26.2335)
  line L642 (33.585, -27.0175) -> (33.585, -26.2335)
  line L643 (32.792, -27.0175) -> (33.585, -27.0175)
  line L644 (30.272, -26.2335) -> (30.272, -27.0175)
  line L645 (31.065, -26.2335) -> (30.272, -26.2335)
  line L646 (31.065, -27.0175) -> (31.065, -26.2335)
  line L647 (30.272, -27.0175) -> (31.065, -27.0175)
  line L648 (27.752, -26.2335) -> (27.752, -27.0175)
  line L649 (28.545, -26.2335) -> (27.752, -26.2335)
  line L650 (28.545, -27.0175) -> (28.545, -26.2335)
  line L651 (27.752, -27.0175) -> (28.545, -27.0175)
  line L652 (25.232, -26.2335) -> (25.232, -27.0175)
  line L653 (26.025, -26.2335) -> (25.232, -26.2335)
  line L654 (26.025, -27.0175) -> (26.025, -26.2335)
  line L655 (25.232, -27.0175) -> (26.025, -27.0175)
  line L656 (22.712, -26.2335) -> (22.712, -27.0175)
  line L657 (23.505, -26.2335) -> (22.712, -26.2335)
  line L658 (23.505, -27.0175) -> (23.505, -26.2335)
  line L659 (22.712, -27.0175) -> (23.505, -27.0175)
  line L660 (20.192, -26.2335) -> (20.192, -27.0175)
  line L661 (20.985, -26.2335) -> (20.192, -26.2335)
  line L662 (20.985, -27.0175) -> (20.985, -26.2335)
  line L663 (20.192, -27.0175) -> (20.985, -27.0175)
  line L664 (17.672, -26.2335) -> (17.672, -27.0175)
  line L665 (18.465, -26.2335) -> (17.672, -26.2335)
  line L666 (18.465, -27.0175) -> (18.465, -26.2335)
  line L667 (17.672, -27.0175) -> (18.465, -27.0175)
  line L668 (15.152, -26.2335) -> (15.152, -27.0175)
  line L669 (15.945, -26.2335) -> (15.152, -26.2335)
  line L670 (15.945, -27.0175) -> (15.945, -26.2335)
  line L671 (15.152, -27.0175) -> (15.945, -27.0175)
  line L672 (12.632, -26.2335) -> (12.632, -27.0175)
  line L673 (13.425, -26.2335) -> (12.632, -26.2335)
  line L674 (13.425, -27.0175) -> (13.425, -26.2335)
  line L675 (12.632, -27.0175) -> (13.425, -27.0175)
  line L676 (10.112, -26.2335) -> (10.112, -27.0175)
  line L677 (10.905, -26.2335) -> (10.112, -26.2335)
  line L678 (10.905, -27.0175) -> (10.905, -26.2335)
  line L679 (10.112, -27.0175) -> (10.905, -27.0175)
  line L680 (7.592, -26.2335) -> (7.592, -27.0175)
  line L681 (8.385, -26.2335) -> (7.592, -26.2335)
  line L682 (8.385, -27.0175) -> (8.385, -26.2335)
  line L683 (7.592, -27.0175) -> (8.385, -27.0175)
  line L684 (5.072, -26.2335) -> (5.072, -27.0175)
  line L685 (5.865, -26.2335) -> (5.072, -26.2335)
  line L686 (5.865, -27.0175) -> (5.865, -26.2335)
  line L687 (5.072, -27.0175) -> (5.865, -27.0175)
  line L688 (2.552, -26.2335) -> (2.552, -27.0175)
  line L689 (3.345, -26.2335) -> (2.552, -26.2335)
  line L690 (3.345, -27.0175) -> (3.345, -26.2335)
  line L691 (2.552, -27.0175) -> (3.345, -27.0175)
  line L692 (0.032, -26.2335) -> (0.032, -27.0175)
  line L693 (0.825, -26.2335) -> (0.032, -26.2335)
  line L694 (0.825, -27.0175) -> (0.825, -26.2335)
  line L695 (0.032, -27.0175) -> (0.825, -27.0175)
  line L696 (-2.488, -26.2335) -> (-2.488, -27.0175)
  line L697 (-1.695, -26.2335) -> (-2.488, -26.2335)
  line L698 (-1.695, -27.0175) -> (-1.695, -26.2335)
  line L699 (-2.488, -27.0175) -> (-1.695, -27.0175)
  line L700 (-5.008, -26.2335) -> (-5.008, -27.0175)
  line L701 (-4.215, -26.2335) -> (-5.008, -26.2335)
  line L702 (-4.215, -27.0175) -> (-4.215, -26.2335)
  line L703 (-5.008, -27.0175) -> (-4.215, -27.0175)
  line L704 (-7.528, -26.2335) -> (-7.528, -27.0175)
  line L705 (-6.735, -26.2335) -> (-7.528, -26.2335)
  line L706 (-6.735, -27.0175) -> (-6.735, -26.2335)
  line L707 (-7.528, -27.0175) -> (-6.735, -27.0175)
  line L708 (-10.048, -26.2335) -> (-10.048, -27.0175)
  line L709 (-9.255, -26.2335) -> (-10.048, -26.2335)
  line L710 (-9.255, -27.0175) -> (-9.255, -26.2335)
  line L711 (-10.048, -27.0175) -> (-9.255, -27.0175)
  line L712 (-12.568, -26.2335) -> (-12.568, -27.0175)
  line L713 (-11.775, -26.2335) -> (-12.568, -26.2335)
  line L714 (-11.775, -27.0175) -> (-11.775, -26.2335)
  line L715 (-12.568, -27.0175) -> (-11.775, -27.0175)
  line L716 (-15.088, -26.2335) -> (-15.088, -27.0175)
  line L717 (-14.295, -26.2335) -> (-15.088, -26.2335)
  line L718 (-14.295, -27.0175) -> (-14.295, -26.2335)
  line L719 (-15.088, -27.0175) -> (-14.295, -27.0175)
  line L720 (45.392, -23.7335) -> (45.392, -24.5175)
  line L721 (46.185, -23.7335) -> (45.392, -23.7335)
  line L722 (46.185, -24.5175) -> (46.185, -23.7335)
  line L723 (45.392, -24.5175) -> (46.185, -24.5175)
  line L724 (42.872, -23.7335) -> (42.872, -24.5175)
  line L725 (43.665, -23.7335) -> (42.872, -23.7335)
  line L726 (43.665, -24.5175) -> (43.665, -23.7335)
  line L727 (42.872, -24.5175) -> (43.665, -24.5175)
  line L728 (40.352, -23.7335) -> (40.352, -24.5175)
  line L729 (41.145, -23.7335) -> (40.352, -23.7335)
  line L730 (41.145, -24.5175) -> (41.145, -23.7335)
  line L731 (40.352, -24.5175) -> (41.145, -24.5175)
  line L732 (37.832, -23.7335) -> (37.832, -24.5175)
  line L733 (38.625, -23.7335) -> (37.832, -23.7335)
  line L734 (38.625, -24.5175) -> (38.625, -23.7335)
  line L735 (37.832, -24.5175) -> (38.625, -24.5175)
  line L736 (35.312, -23.7335) -> (35.312, -24.5175)
  line L737 (36.105, -23.7335) -> (35.312, -23.7335)
  line L738 (36.105, -24.5175) -> (36.105, -23.7335)
  line L739 (35.312, -24.5175) -> (36.105, -24.5175)
  line L740 (32.792, -23.7335) -> (32.792, -24.5175)
  line L741 (33.585, -23.7335) -> (32.792, -23.7335)
  line L742 (33.585, -24.5175) -> (33.585, -23.7335)
  line L743 (32.792, -24.5175) -> (33.585, -24.5175)
  line L744 (30.272, -23.7335) -> (30.272, -24.5175)
  line L745 (31.065, -23.7335) -> (30.272, -23.7335)
  line L746 (31.065, -24.5175) -> (31.065, -23.7335)
  line L747 (30.272, -24.5175) -> (31.065, -24.5175)
  line L748 (27.752, -23.7335) -> (27.752, -24.5175)
  line L749 (28.545, -23.7335) -> (27.752, -23.7335)
  line L750 (28.545, -24.5175) -> (28.545, -23.7335)
  line L751 (27.752, -24.5175) -> (28.545, -24.5175)
  line L752 (25.232, -23.7335) -> (25.232, -24.5175)
  line L753 (26.025, -23.7335) -> (25.232, -23.7335)
  line L754 (26.025, -24.5175) -> (26.025, -23.7335)
  line L755 (25.232, -24.5175) -> (26.025, -24.5175)
  line L756 (22.712, -23.7335) -> (22.712, -24.5175)
  line L757 (23.505, -23.7335) -> (22.712, -23.7335)
  line L758 (23.505, -24.5175) -> (23.505, -23.7335)
  line L759 (22.712, -24.5175) -> (23.505, -24.5175)
  line L760 (20.192, -23.7335) -> (20.192, -24.5175)
  line L761 (20.985, -23.7335) -> (20.192, -23.7335)
  line L762 (20.985, -24.5175) -> (20.985, -23.7335)
  line L763 (20.192, -24.5175) -> (20.985, -24.5175)
  line L764 (17.672, -23.7335) -> (17.672, -24.5175)
  line L765 (18.465, -23.7335) -> (17.672, -23.7335)
  line L766 (18.465, -24.5175) -> (18.465, -23.7335)
  line L767 (17.672, -24.5175) -> (18.465, -24.5175)
  line L768 (15.152, -23.7335) -> (15.152, -24.5175)
  line L769 (15.945, -23.7335) -> (15.152, -23.7335)
  line L770 (15.945, -24.5175) -> (15.945, -23.7335)
  line L771 (15.152, -24.5175) -> (15.945, -24.5175)
  line L772 (12.632, -23.7335) -> (12.632, -24.5175)
  line L773 (13.425, -23.7335) -> (12.632, -23.7335)
  line L774 (13.425, -24.5175) -> (13.425, -23.7335)
  line L775 (12.632, -24.5175) -> (13.425, -24.5175)
  line L776 (10.112, -23.7335) -> (10.112, -24.5175)
  line L777 (10.905, -23.7335) -> (10.112, -23.7335)
  line L778 (10.905, -24.5175) -> (10.905, -23.7335)
  line L779 (10.112, -24.5175) -> (10.905, -24.5175)
  line L780 (7.592, -23.7335) -> (7.592, -24.5175)
  line L781 (8.385, -23.7335) -> (7.592, -23.7335)
  line L782 (8.385, -24.5175) -> (8.385, -23.7335)
  line L783 (7.592, -24.5175) -> (8.385, -24.5175)
  line L784 (5.072, -23.7335) -> (5.072, -24.5175)
  line L785 (5.865, -23.7335) -> (5.072, -23.7335)
  line L786 (5.865, -24.5175) -> (5.865, -23.7335)
  line L787 (5.072, -24.5175) -> (5.865, -24.5175)
  line L788 (2.552, -23.7335) -> (2.552, -24.5175)
  line L789 (3.345, -23.7335) -> (2.552, -23.7335)
  line L790 (3.345, -24.5175) -> (3.345, -23.7335)
  line L791 (2.552, -24.5175) -> (3.345, -24.5175)
  line L792 (0.032, -23.7335) -> (0.032, -24.5175)
  line L793 (0.825, -23.7335) -> (0.032, -23.7335)
  line L794 (0.825, -24.5175) -> (0.825, -23.7335)
  line L795 (0.032, -24.5175) -> (0.825, -24.5175)
  line L796 (-2.488, -23.7335) -> (-2.488, -24.5175)
  line L797 (-1.695, -23.7335) -> (-2.488, -23.7335)
  line L798 (-1.695, -24.5175) -> (-1.695, -23.7335)
  line L799 (-2.488, -24.5175) -> (-1.695, -24.5175)
  line L800 (-5.008, -23.7335) -> (-5.008, -24.5175)
  line L801 (-4.215, -23.7335) -> (-5.008, -23.7335)
  line L802 (-4.215, -24.5175) -> (-4.215, -23.7335)
  line L803 (-5.008, -24.5175) -> (-4.215, -24.5175)
  line L804 (-7.528, -23.7335) -> (-7.528, -24.5175)
  line L805 (-6.735, -23.7335) -> (-7.528, -23.7335)
  line L806 (-6.735, -24.5175) -> (-6.735, -23.7335)
  line L807 (-7.528, -24.5175) -> (-6.735, -24.5175)
  line L808 (-10.048, -23.7335) -> (-10.048, -24.5175)
  line L809 (-9.255, -23.7335) -> (-10.048, -23.7335)
  line L810 (-9.255, -24.5175) -> (-9.255, -23.7335)
  line L811 (-10.048, -24.5175) -> (-9.255, -24.5175)
  line L812 (-12.568, -23.7335) -> (-12.568, -24.5175)
  line L813 (-11.775, -23.7335) -> (-12.568, -23.7335)
  line L814 (-11.775, -24.5175) -> (-11.775, -23.7335)
  line L815 (-12.568, -24.5175) -> (-11.775, -24.5175)
  line L816 (-15.088, -23.7335) -> (-15.088, -24.5175)
  line L817 (-14.295, -23.7335) -> (-15.088, -23.7335)
  line L818 (-14.295, -24.5175) -> (-14.295, -23.7335)
  line L819 (-15.088, -24.5175) -> (-14.295, -24.5175)
  line L820 (47.0585, -27.8955) -> (-15.9615, -27.8955)
  line L821 (-15.9615, -27.8955) -> (-15.9615, -22.8555)
  line L822 (-15.9615, -22.8555) -> (47.0585, -22.8555)
  line L823 (47.0585, -22.8555) -> (47.0585, -27.8955)
  point P0 (0, 0)
  point P1 (45.7885, 33.5405)
  point P2 (45.7885, 26.6255)
  point P3 (45.7885, 31.0405)
  point P4 (45.7885, 24.1255)
  point P5 (-14.6915, 26.6255)
  point P6 (45.7885, -33.5405)
  point P7 (45.7885, -26.6255)
  point P8 (45.7885, -31.0405)
  point P9 (45.7885, -24.1255)
  point P10 (-14.6915, -26.6255)
  dimension "d0" = 107.193
  dimension "d1" = 75.991
  dimension "d2" = 2
  dimension "d3" = 2
  dimension "d4" = 2
  dimension "d5" = 2
  dimension "d6" = 3
  dimension "d7" = 3
  dimension "d8" = 3
  dimension "d9" = 3
  dimension "d10" = 3
  dimension "d11" = 3
  dimension "d12" = 3
  dimension "d13" = 3
  dimension "d16" = 0.793
  dimension "d17" = 0.784
  dimension "d18" = 4.808
  dimension "d19" = 1.455
  dimension "d22" = 2.52
  dimension "d25" = 2.5
  dimension "d28" = 0.784
  dimension "d29" = 4.415
  dimension "d32" = 2.52
  dimension "d35" = 2.5
  dimension "d38" = 1.27
  dimension "d39" = 1.27
  dimension "d40" = 1.27
  dimension "d41" = 1.27
  constraints: 1648 end point, 10 midpoint, 8 parallel, 7 horizontal, 4 centre point, 4 perpendicular, 3 vertical, 787 other
  measures "d0" distance of L2.end L1.end
  measures "d1" distance of L1.end L0.end
  measures "d2" diameter of A0
  measures "d3" diameter of A1
  measures "d4" diameter of A2
  measures "d5" diameter of A3
  measures "d6" distance from line of L0 A2.centre
  measures "d7" distance from line of L1 A2.centre
  measures "d8" distance from line of L2 A3.centre
  measures "d9" distance from line of L1 A3.centre
  measures "d10" distance from line of A0.centre L0
  measures "d11" distance from line of L3 A0.centre
  measures "d12" distance from line of L2 A1.centre
  measures "d13" distance from line of L3 A1.centre
  measures "d16" distance of L8.end L7.end
  measures "d17" distance of L7.end L6.end
  measures "d18" horizontal distance of A0.centre point (45.788, 33.541)
  measures "d19" vertical distance of point (45.788, 33.541) A0.centre
  measures "d22" distance of L6.end L13.start
  measures "d25" distance of L6.end L109.start
  measures "d28" distance of L208.end L209.end
  measures "d29" distance of point (45.788, 26.626) point (45.788, 31.041)
  measures "d32" distance of L210.end L217.start
  measures "d35" distance of L210.end L313.start
  measures "d38" distance from line of L410 point (45.788, 26.626)
  measures "d39" distance from line of L413 point (45.788, 26.626)
  measures "d40" distance from line of L412 point (45.788, 24.126)
  measures "d41" distance from line of L411 point (-14.692, 26.626)
extrude "Extrusion2" add sketch "Sketch1" along normal blind 2 contours L3 L2 L1 L0
extrude "Extrusion3" add sketch "Sketch1" along normal blind 11.5 contours L9 L8 L7 L6
pattern_linear "Rectangular Pattern1" count 25 spacing 2.52 along (1, 0, 0) count 2 spacing 2.5 along (0, 0, -1) of "Extrusion3"
extrude "Extrusion4" add sketch "Sketch1" against normal blind 7 contours L413 L412 L411 L410
mirror "Mirror1" about plane through (0, 0, 0) normal (0, 0, 1) of "Extrusion4", "Extrusion3", "Rectangular Pattern1"
sketch "Sketch2" plane through (0, 2, 0) normal (0, 1, 0) x (1, 0, 0)
  line L0 (-47.0585, -22.8555) -> (15.9615, -22.8555) projected
  line L1 (-47.0585, -27.8955) -> (-47.0585, -22.8555) projected
  line L2 (15.9615, -27.8955) -> (-47.0585, -27.8955) projected
  line L3 (15.9615, -22.8555) -> (15.9615, -27.8955) projected
  line L4 (15.9615, 27.8955) -> (15.9615, 22.8555) projected
  line L5 (-47.0585, 27.8955) -> (15.9615, 27.8955) projected
  line L6 (15.9615, 22.8555) -> (-47.0585, 22.8555) projected
  line L7 (-47.0585, 22.8555) -> (-47.0585, 27.8955) projected
  point P0 (0, 0)
extrude "Extrusion5" add sketch "Sketch2" against normal blind 2
sketch "Sketch3" plane through (0, 2, 0) normal (0, 1, 0) x (1, 0, 0)
  line L0 (-46.185, -33.9325) -> (-45.392, -33.9325) projected
  line L1 (-45.392, -33.9325) -> (-45.392, -33.1485) projected
  line L2 (-45.392, -33.1485) -> (-46.185, -33.1485) projected
  line L3 (-46.185, -33.1485) -> (-46.185, -33.9325) projected
  line L4 (15.979, -34.2905) -> (-47.021, -34.2905)
  line L5 (-47.021, -34.2905) -> (-47.021, -30.2905)
  line L6 (-47.021, -30.2905) -> (15.979, -30.2905)
  line L7 (15.979, -30.2905) -> (15.979, -34.2905)
  line L8 (-46.185, -31.4325) -> (-45.392, -31.4325) projected
  line L9 (-45.392, -31.4325) -> (-45.392, -30.6485) projected
  line L10 (-45.392, -30.6485) -> (-46.185, -30.6485) projected
  line L11 (-46.185, -30.6485) -> (-46.185, -31.4325) projected
  line L12 (-2, 0) -> (2, 0)
  line L13 (15.979, 34.2905) -> (-47.021, 34.2905)
  line L14 (-47.021, 34.2905) -> (-47.021, 30.2905)
  line L15 (-47.021, 30.2905) -> (15.979, 30.2905)
  line L16 (15.979, 30.2905) -> (15.979, 34.2905)
  point P0 (0, 0)
  dimension "d56" = 63
  dimension "d57" = 4
  dimension "d58" = 0.836
  dimension "d59" = 0.358
  constraints: 18 end point, 4 symmetric about line, 2 horizontal, 2 parallel, 1 perpendicular
  measures "d56" distance of L5.end L6.end
  measures "d57" distance of L4.end L5.end
  measures "d58" distance between parallel lines of L5 L3
  measures "d59" distance between parallel lines of L4 L0
extrude "Extrusion6" add sketch "Sketch3" along normal blind 2.5
sketch "Sketch4" plane through (0, 2, 0) normal (0, 1, 0) x (1, 0, 0)
  line L0 (-50.6925, -27) -> (51, -27)
  line L1 (51, -27) -> (51, 28.0529)
  line L2 (51, 28.0529) -> (-50.6925, 28.0529)
  line L3 (-50.6925, 28.0529) -> (-50.6925, -27)
  point P0 (0, 0)
  constraints: 8 end point, 2 parallel, 1 horizontal, 1 perpendicular
extrude "Extrusion7" add sketch "Sketch4" along normal blind 21.26
sketch "Sketch5" plane through (0, 23.26, 0) normal (0, 1, 0) x (1, 0, 0)
  line L0 (-38.1721, 15.9736) -> (13.2473, 15.9736) construction
  line L1 (13.2473, 15.9736) -> (13.2473, 12.3261) construction
  line L2 (13.2473, 12.3261) -> (-38.1721, 12.3261) construction
  line L3 (-38.1721, 12.3261) -> (-38.1721, 15.9736) construction
  point P0 (0, 0)
  constraints: 2 other
body "Solid2"
